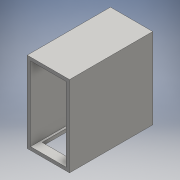
# Autodesk Inventor part: Riight Leg
Saved by Autodesk Inventor 2016 (Build 200138000, 138)
## iProperties
Created: 2017-05-09
Part Number: Riight Leg
Material: Generic
Document SubType Name: Modeling
Designer: M220404
Density: 1 g/cm^3
Appearance: Default
Author: M220404
Autodesk Inventor part; units mm, degrees
ref_plane "YZ Plane" through (0, 0, 0) normal (1, 0, 0) x (0, 1, 0)
ref_plane "XZ Plane" through (0, 0, 0) normal (0, 1, 0) x (-1, 0, 0)
ref_plane "XY Plane" through (0, 0, 0) normal (0, 0, 1) x (1, 0, 0)
sketch "Sketch1" plane through (0, 0, 0) normal (0, 1, 0) x (-1, 0, 0)
  line L0 (0, 0) -> (-250, 0)
  line L1 (-250, 0) -> (-250, -520)
  line L2 (-250, -520) -> (0, -520)
  line L3 (0, -520) -> (0, 0)
  line L4 (23, -543) -> (-273, -543)
  line L5 (-273, -543) -> (-273, 23)
  line L6 (-273, 23) -> (23, 23)
  line L7 (23, 23) -> (23, -543)
  dimension "d0" = 250
  dimension "d1" = 520
  dimension "d2" = 23
  constraints: 16 end point, 4 parallel, 2 perpendicular, 1 horizontal, 3 other
  measures "d0" distance of L2.end L1.end
  measures "d1" distance of L1.end L0.end
  measures "d2" distance between parallel lines of L2 L4
extrude "Extrusion1" add sketch "Sketch1" along normal blind 583
sketch "Sketch2" plane through (273, 0, -543) normal (0, 0, -1) x (-1, 0, 0)
  line L0 (38, 506) -> (258, 506)
  line L1 (258, 506) -> (258, 66)
  line L2 (258, 66) -> (38, 66)
  line L3 (38, 66) -> (38, 506)
  line L4 (0, 583) -> (296, 583) projected
  line L5 (296, 0) -> (296, 583) projected
  point P0 (273, 0)
  dimension "d5" = 220
  dimension "d6" = 440
  dimension "d7" = 77
  dimension "d8" = 38
  constraints: 8 end point, 2 parallel, 1 horizontal, 1 perpendicular
  measures "d5" distance of L1.end L2.end
  measures "d6" distance of L0.end L1.end
  measures "d7" distance between parallel lines of L4 L0
  measures "d8" distance between parallel lines of L5 L1
extrude "Extrusion2" cut sketch "Sketch2" against normal up to surface (23 mm away)
sketch "Sketch3" plane through (-23, 0, -543) normal (-1, 0, 0) x (0, 0, 1)
  line L0 (143, 510) -> (213, 510)
  line L1 (213, 510) -> (213, 430)
  line L2 (213, 430) -> (143, 430)
  line L3 (143, 430) -> (143, 510)
  line L4 (566, 0) -> (0, 0) projected
  line L5 (0, 0) -> (0, 583) projected
  point P0 (543, 0)
  dimension "d11" = 70
  dimension "d12" = 80
  dimension "d13" = 430
  dimension "d14" = 143
  constraints: 8 end point, 2 parallel, 1 horizontal, 1 perpendicular
  measures "d11" distance of L1.end L2.end
  measures "d12" distance of L0.end L1.end
  measures "d13" distance between parallel lines of L4 L2
  measures "d14" distance between parallel lines of L5 L3
extrude "Extrusion3" cut sketch "Sketch3" against normal up to surface (23 mm away)
sketch "Sketch4" plane through (0, 583, 0) normal (0, 1, 0) x (1, 0, 0)
  point P0 (0, 0)
sketch "Sketch5" plane through (0, 583, 0) normal (0, 1, 0) x (1, 0, 0)
  line L0 (250, 0) -> (250, 520) projected
  line L1 (250, 520) -> (0, 520) projected
  line L2 (250, 0) -> (0, 0)
  line L3 (0, 0) -> (0, 520)
  line L4 (0, 520) -> (250, 520)
  line L5 (250, 520) -> (250, 0)
  line L6 (47, 47) -> (203, 47)
  line L7 (203, 47) -> (203, 473)
  line L8 (203, 473) -> (47, 473)
  line L9 (47, 473) -> (47, 47)
  dimension "d17" = 47
  constraints: 16 end point, 4 parallel, 2 perpendicular, 1 horizontal, 3 other
  measures "d17" distance between parallel lines of L2 L6
extrude "Extrusion4" add sketch "Sketch5" against normal up to surface (73 mm away)
sketch "Sketch6" plane through (0, 583, 0) normal (0, 1, 0) x (1, 0, 0)
  circle A0 centre (228, 373) radius 8
  line L0 (273, 543) -> (-23, 543) projected
  line L1 (273, -23) -> (273, 543) projected
  circle A1 centre (228, 147) radius 8
  line L2 (-23, -23) -> (273, -23) projected
  line L3 (125, -23) -> (125, 543) construction
  circle A2 centre (22, 373) radius 8
  circle A3 centre (22, 147) radius 8
  point P0 (0, 0)
  dimension "d20" = 16
  dimension "d21" = 170
  dimension "d22" = 45
  dimension "d23" = 16
  dimension "d24" = 170
  dimension "d25" = 45
  constraints: 4 centre point, 2 end point, 2 midpoint, 2 symmetric about line, 2 other
  measures "d20" diameter of A0
  measures "d21" distance from line of L0 A0.centre
  measures "d22" distance from line of L1 A0.centre
  measures "d23" diameter of A1
  measures "d24" distance from line of L2 A1.centre
  measures "d25" distance from line of L1 A1.centre
extrude "Extrusion5" cut sketch "Sketch6" against normal blind 10
body "Solid1"
